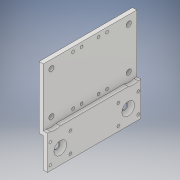
# Autodesk Inventor part: КВ33.044.201
Saved by Autodesk Inventor 2019 (Build 230136000, 136)
## iProperties
Created: 2019-07-15
Part Number: КВ33.044.201
Material: Пластик АБС
Document SubType Name: Modeling
Designer: Петров Иван
Density: 1.06 g/cm^3
Appearance: Гладкий — белый
Description: Щека каретки
Mass: 64.5472 g
Surface Area: 280.738 cm^2
Volume: 60.8936 cm^3
Author: Петров Иван
Autodesk Inventor part; units mm, degrees
(part 1 of 3)
ref_plane "YZ Plane" through (0, 0, 0) normal (1, 0, 0) x (0, 1, 0)
ref_plane "XZ Plane" through (0, 0, 0) normal (0, 1, 0) x (-1, 0, 0)
ref_plane "XY Plane" through (0, 0, 0) normal (0, 0, 1) x (1, 0, 0)
sketch "Эскиз1" plane through (0, 0, 0) normal (1, 0, 0) x (0, 1, 0)
  line L0 (34, 15) -> (34, -15)
  line L1 (-34, -15) -> (-34, 15)
  line L2 (-34, 15) -> (-34, 55)
  line L3 (-34, 55) -> (34, 55)
  line L4 (34, 55) -> (34, 15)
  line L5 (-34, -15) -> (-34, -55)
  line L6 (-34, -55) -> (34, -55)
  line L7 (34, -55) -> (34, -15)
  line L8 (34, 55) -> (24.5, 55)
  line L9 (24.5, 55) -> (24.5, 45.5)
  line L10 (27.5, 45.5) -> (34, 45.5)
  line L11 (34, 45.5) -> (34, 55)
  line L12 (-34, 55) -> (-24.5, 55)
  line L13 (-24.5, 55) -> (-24.5, 45.5)
  line L14 (-27.5, 45.5) -> (-34, 45.5)
  line L15 (-34, 45.5) -> (-34, 55)
  line L16 (-34, -55) -> (-24.5, -55)
  line L17 (-24.5, -55) -> (-24.5, -45.5)
  line L18 (-27.5, -45.5) -> (-34, -45.5)
  line L19 (-34, -45.5) -> (-34, -55)
  line L20 (34, -55) -> (24.5, -55)
  line L21 (24.5, -55) -> (24.5, -45.5)
  line L22 (27.5, -45.5) -> (34, -45.5)
  line L23 (34, -45.5) -> (34, -55)
  circle A0 centre (24.5, 45.5) radius 3
  circle A1 centre (-24.5, 45.5) radius 3
  circle A2 centre (-24.5, -45.5) radius 3
  circle A3 centre (24.5, -45.5) radius 3
  line L24 (34, 55) -> (-34, 55)
  line L25 (-34, 55) -> (-34, -55)
  line L26 (-34, -55) -> (34, -55)
  line L27 (34, -55) -> (34, 55)
  point P0 (0, 0)
  dimension "d12" = 6
  dimension "d13" = 6
  dimension "d14" = 6
  dimension "d15" = 6
  dimension "d4" = 9.5
  dimension "d5" = 9.5
  dimension "d6" = 9.5
  dimension "d7" = 9.5
  dimension "d8" = 9.5
  dimension "d9" = 9.5
  dimension "d10" = 9.5
  dimension "d11" = 9.5
  constraints: 56 end point, 13 parallel, 7 horizontal, 5 perpendicular, 5 vertical, 4 coincident, 4 horizontal alignment, 1 point on line, 8 other
  measures "d4" distance of L10.end L9.end
  measures "d5" distance of L9.end L8.end
  measures "d6" distance of L13.end L14.end
  measures "d7" distance of L12.end L13.end
  measures "d8" distance of L16.end L17.end
  measures "d9" distance of L17.end L18.end
  measures "d10" distance of L20.end L21.end
  measures "d11" distance of L21.end L22.end
extrude "Выдавливание1" add sketch "Эскиз1" along normal blind 5 contours L0 L7 L22 A3 L21 L6 L17 A2 L18 L5 L1 L2 L14 A1 L13 L3 L9 A0 L10 L4 | L10 A0 L9 L3 L4 | L7 L6 L21 A3 L22 | L13 A1 L14 L2 L3 | L6 L5 L18 A2 L17
sketch "Эскиз2" plane through (0, -34, -55) normal (0, -1, 0) x (1, 0, 0)
  line L0 (0, 110) -> (5, 110) projected
  line L1 (0, 110) -> (10, 110)
  line L2 (10, 110) -> (10, 0)
  line L3 (10, 0) -> (0, 0)
  line L4 (0, 0) -> (0, 110)
  point P0 (0, 55)
  dimension "d18" = 10
  dimension "d19" = 110
  constraints: 8 end point, 2 parallel, 1 horizontal, 1 perpendicular
  measures "d18" distance of L2.end L3.end
  measures "d19" distance of L1.end L2.end
extrude "Выдавливание2" add sketch "Эскиз2" along normal blind 5
sketch "Эскиз3" plane through (0, -39, -55) normal (0, -1, 0) x (1, 0, 0)
  line L0 (10, 0) -> (10, 110) projected
  line L1 (5, 0) -> (5, 110) projected
  line L2 (10, 110) -> (5, 110)
  line L3 (5, 110) -> (5, 0)
  line L4 (5, 0) -> (10, 0)
  line L5 (10, 0) -> (10, 110)
  point P0 (0, 55)
  constraints: 8 end point, 2 parallel, 1 horizontal, 1 perpendicular
extrude "Выдавливание3" add sketch "Эскиз3" along normal blind 35
sketch "Эскиз4" plane through (5, -39, -55) normal (-1, 0, 0) x (0, 0, 1)
  arc A0 (18.9646, -11.5001) -> (20.0253, -11.0608) centre (18.9646, -10.0001) ccw
  line L0 (18.9646, -11.5001) -> (15.7747, -11.5001)
  line L1 (15.7747, -11.5001) -> (15.0002, -12.15)
  line L2 (15.0002, -12.15) -> (14.2254, -11.4999)
  line L3 (14.2254, -11.4999) -> (11.0358, -11.4999)
  arc A1 (9.9751, -11.0606) -> (11.0358, -11.4999) centre (11.0358, -9.9999) ccw
  line L4 (9.9751, -11.0606) -> (6.6464, -7.7319)
  arc A2 (6.5, -7.3783) -> (6.6464, -7.7319) centre (7, -7.3783) ccw
  line L5 (6.5, -7.3783) -> (6.5, -4.9)
  arc A3 (6.7, -4.7) -> (6.5, -4.9) centre (6.7, -4.9) ccw
  line L6 (6.7, -4.7) -> (10.7, -4.7)
  arc A4 (10.7, -4.7) -> (10.9, -4.5) centre (10.7, -4.5) ccw
  line L7 (10.9, -4.5) -> (10.9, -3.4)
  arc A5 (10.9, -3.4) -> (10.7, -3.2) centre (10.7, -3.4) ccw
  line L8 (10.7, -3.2) -> (10.3, -3.2)
  line L9 (10.3, -3.2) -> (10.3, -2.6999)
  arc A6 (10.3, -2.6999) -> (10.0999, -2.4999) centre (10.0999, -2.6999) ccw
  line L10 (10.0999, -2.4999) -> (1.5, -2.4999)
  arc A7 (1.5, -2.4999) -> (0, -3.9999) centre (1.5, -3.9999) ccw
  line L11 (0, -3.9999) -> (0, -12.6001)
  arc A8 (0, -12.6001) -> (0.2, -12.8001) centre (0.2, -12.6001) ccw
  line L12 (0.2, -12.8001) -> (0.7, -12.8001)
  line L13 (0.7, -12.8001) -> (0.7, -13.2001)
  arc A9 (0.7, -13.2001) -> (0.9, -13.4001) centre (0.9, -13.2001) ccw
  line L14 (0.9, -13.4001) -> (2, -13.4001)
  arc A10 (2, -13.4001) -> (2.2, -13.2001) centre (2, -13.2001) ccw
  line L15 (2.2, -13.2001) -> (2.2, -9.2)
  arc A11 (2.4, -9) -> (2.2, -9.2) centre (2.4, -9.2) ccw
  line L16 (2.4, -9) -> (4.8789, -9)
  arc A12 (5.2325, -9.1464) -> (4.8789, -9) centre (4.8789, -9.5) ccw
  line L17 (5.2325, -9.1464) -> (8.5608, -12.4747)
  arc A13 (9.0001, -13.5354) -> (8.5608, -12.4747) centre (7.5001, -13.5354) ccw
  line L18 (9.0001, -13.5354) -> (9.0001, -16.7253)
  line L19 (9.0001, -16.7253) -> (9.65, -17.4998)
  line L20 (9.65, -17.4998) -> (8.9999, -18.2746)
  line L21 (8.9999, -18.2746) -> (8.9999, -21.4642)
  arc A14 (8.5606, -22.5249) -> (8.9999, -21.4642) centre (7.4999, -21.4642) ccw
  line L22 (8.5606, -22.5249) -> (5.2319, -25.8536)
  arc A15 (4.8783, -26) -> (5.2319, -25.8536) centre (4.8783, -25.5) ccw
  line L23 (4.8783, -26) -> (2.4, -26)
  arc A16 (2.2, -25.8) -> (2.4, -26) centre (2.4, -25.8) ccw
  line L24 (2.2, -25.8) -> (2.2, -21.8)
  arc A17 (2.2, -21.8) -> (2, -21.6) centre (2, -21.8) ccw
  line L25 (2, -21.6) -> (0.9, -21.6)
  arc A18 (0.9, -21.6) -> (0.7, -21.8) centre (0.9, -21.8) ccw
  line L26 (0.7, -21.8) -> (0.7, -22.2)
  line L27 (0.7, -22.2) -> (0.2, -22.2)
  arc A19 (0.2, -22.2) -> (0, -22.4) centre (0.2, -22.4) ccw
  line L28 (0, -22.4) -> (0, -31)
  arc A20 (0, -31) -> (1.5, -32.5) centre (1.5, -31) ccw
  line L29 (1.5, -32.5) -> (10.1002, -32.5)
  arc A21 (10.1002, -32.5) -> (10.3002, -32.3) centre (10.1002, -32.3) ccw
  line L30 (10.3002, -32.3) -> (10.3002, -31.8)
  line L31 (10.3002, -31.8) -> (10.7002, -31.8)
  arc A22 (10.7002, -31.8) -> (10.9002, -31.6) centre (10.7002, -31.6) ccw
  line L32 (10.9002, -31.6) -> (10.9002, -30.5)
  arc A23 (10.9002, -30.5) -> (10.7002, -30.3) centre (10.7002, -30.5) ccw
  line L33 (10.7002, -30.3) -> (6.7001, -30.3)
  arc A24 (6.5001, -30.1) -> (6.7001, -30.3) centre (6.7001, -30.1) ccw
  line L34 (6.5001, -30.1) -> (6.5001, -27.6211)
  arc A25 (6.6466, -27.2675) -> (6.5001, -27.6211) centre (7.0001, -27.6211) ccw
  line L35 (6.6466, -27.2675) -> (9.9749, -23.9392)
  arc A26 (11.0355, -23.4999) -> (9.9749, -23.9392) centre (11.0355, -24.9999) ccw
  line L36 (11.0355, -23.4999) -> (14.2255, -23.4999)
  line L37 (14.2255, -23.4999) -> (15, -22.85)
  line L38 (15, -22.85) -> (15.7747, -23.5001)
  line L39 (15.7747, -23.5001) -> (18.9644, -23.5001)
  arc A27 (20.025, -23.9394) -> (18.9644, -23.5001) centre (18.9644, -25.0001) ccw
  line L40 (20.025, -23.9394) -> (23.3537, -27.2681)
  arc A28 (23.5001, -27.6217) -> (23.3537, -27.2681) centre (23.0001, -27.6217) ccw
  line L41 (23.5001, -27.6217) -> (23.5001, -30.1)
  arc A29 (23.3001, -30.3) -> (23.5001, -30.1) centre (23.3001, -30.1) ccw
  line L42 (23.3001, -30.3) -> (19.3002, -30.3)
  arc A30 (19.3002, -30.3) -> (19.1002, -30.5) centre (19.3002, -30.5) ccw
  line L43 (19.1002, -30.5) -> (19.1002, -31.6)
  arc A31 (19.1002, -31.6) -> (19.3002, -31.8) centre (19.3002, -31.6) ccw
  line L44 (19.3002, -31.8) -> (19.7002, -31.8)
  line L45 (19.7002, -31.8) -> (19.7002, -32.3)
  arc A32 (19.7002, -32.3) -> (19.9002, -32.5) centre (19.9002, -32.3) ccw
  line L46 (19.9002, -32.5) -> (28.5001, -32.5)
  arc A33 (28.5001, -32.5) -> (30.0001, -31) centre (28.5001, -31) ccw
  line L47 (30.0001, -31) -> (30.0001, -22.3998)
  arc A34 (30.0001, -22.3998) -> (29.8001, -22.1998) centre (29.8001, -22.3998) ccw
  line L48 (29.8001, -22.1998) -> (29.3001, -22.1998)
  line L49 (29.3001, -22.1998) -> (29.3001, -21.7998)
  arc A35 (29.3001, -21.7998) -> (29.1001, -21.5998) centre (29.1001, -21.7998) ccw
  line L50 (29.1001, -21.5998) -> (28.0001, -21.5998)
  arc A36 (28.0001, -21.5998) -> (27.8001, -21.7998) centre (28.0001, -21.7998) ccw
  line L51 (27.8001, -21.7998) -> (27.8001, -25.7999)
  arc A37 (27.6001, -25.9999) -> (27.8001, -25.7999) centre (27.6001, -25.7999) ccw
  line L52 (27.6001, -25.9999) -> (25.1212, -25.9999)
  arc A38 (24.7677, -25.8534) -> (25.1212, -25.9999) centre (25.1212, -25.4999) ccw
  line L53 (24.7677, -25.8534) -> (21.4394, -22.5251)
  arc A39 (21, -21.4645) -> (21.4394, -22.5251) centre (22.5, -21.4645) ccw
  line L54 (21, -21.4645) -> (21, -18.2745)
  line L55 (21, -18.2745) -> (20.3501, -17.5)
  line L56 (20.3501, -17.5) -> (21.0002, -16.7253)
  line L57 (21.0002, -16.7253) -> (21.0002, -13.5356)
  arc A40 (21.4396, -12.475) -> (21.0002, -13.5356) centre (22.5002, -13.5356) ccw
  line L58 (21.4396, -12.475) -> (24.7682, -9.1463)
  arc A41 (25.1218, -8.9999) -> (24.7682, -9.1463) centre (25.1218, -9.4999) ccw
  line L59 (25.1218, -8.9999) -> (27.6001, -8.9999)
  arc A42 (27.8001, -9.1999) -> (27.6001, -8.9999) centre (27.6001, -9.1999) ccw
  line L60 (27.8001, -9.1999) -> (27.8001, -13.1998)
  arc A43 (27.8001, -13.1998) -> (28.0001, -13.3998) centre (28.0001, -13.1998) ccw
  line L61 (28.0001, -13.3998) -> (29.1001, -13.3998)
  arc A44 (29.1001, -13.3998) -> (29.3001, -13.1998) centre (29.1001, -13.1998) ccw
  line L62 (29.3001, -13.1998) -> (29.3001, -12.7999)
  line L63 (29.3001, -12.7999) -> (29.8001, -12.7999)
  arc A45 (29.8001, -12.7999) -> (30.0001, -12.5999) centre (29.8001, -12.5999) ccw
  line L64 (30.0001, -12.5999) -> (30.0001, -3.9998)
  arc A46 (30.0001, -3.9998) -> (28.5001, -2.4998) centre (28.5001, -3.9998) ccw
  line L65 (28.5001, -2.4998) -> (19.8999, -2.4998)
  arc A47 (19.8999, -2.4998) -> (19.6999, -2.6998) centre (19.8999, -2.6998) ccw
  line L66 (19.6999, -2.6998) -> (19.6999, -3.2)
  line L67 (19.6999, -3.2) -> (19.2999, -3.2)
  arc A48 (19.2999, -3.2) -> (19.0999, -3.4) centre (19.2999, -3.4) ccw
  line L68 (19.0999, -3.4) -> (19.0999, -4.5)
  arc A49 (19.0999, -4.5) -> (19.2999, -4.7) centre (19.2999, -4.5) ccw
  line L69 (19.2999, -4.7) -> (23.3, -4.7)
  arc A50 (23.5, -4.9) -> (23.3, -4.7) centre (23.3, -4.9) ccw
  line L70 (23.5, -4.9) -> (23.5, -7.3789)
  arc A51 (23.3536, -7.7325) -> (23.5, -7.3789) centre (23, -7.3789) ccw
  line L71 (23.3536, -7.7325) -> (20.0253, -11.0608)
  arc A52 (2.2887, -27.7413) -> (2.5454, -27.8134) centre (2.4574, -27.6338) ccw
  arc A53 (3.9543, -27.8134) -> (2.5454, -27.8134) centre (3.2499, -29.25) ccw
  arc A54 (3.9543, -27.8134) -> (4.211, -27.7413) centre (4.0423, -27.6338) ccw
  line L72 (4.3695, -27.4925) -> (4.211, -27.7413)
  arc A55 (4.5382, -27.4) -> (4.3695, -27.4925) centre (4.5382, -27.6) ccw
  line L73 (4.6999, -27.4) -> (4.5382, -27.4)
  arc A56 (5.0999, -27.8) -> (4.6999, -27.4) centre (4.6999, -27.8) ccw
  line L74 (5.0999, -27.9617) -> (5.0999, -27.8)
  arc A57 (5.0073, -28.1304) -> (5.0999, -27.9617) centre (4.8999, -27.9617) ccw
  line L75 (4.7586, -28.2888) -> (5.0073, -28.1304)
  arc A58 (4.7586, -28.2888) -> (4.6864, -28.5456) centre (4.866, -28.4575) ccw
  arc A59 (4.6864, -29.9544) -> (4.6864, -28.5456) centre (3.2499, -29.25) ccw
  arc A60 (4.6864, -29.9544) -> (4.7586, -30.2111) centre (4.866, -30.0425) ccw
  line L76 (5.0073, -30.3696) -> (4.7586, -30.2111)
  arc A61 (5.0999, -30.5383) -> (5.0073, -30.3696) centre (4.8999, -30.5383) ccw
  line L77 (5.0999, -30.7) -> (5.0999, -30.5383)
  arc A62 (4.6999, -31.1) -> (5.0999, -30.7) centre (4.6999, -30.7) ccw
  line L78 (4.5382, -31.1) -> (4.6999, -31.1)
  arc A63 (4.3695, -31.0075) -> (4.5382, -31.1) centre (4.5382, -30.9) ccw
  line L79 (4.211, -30.7587) -> (4.3695, -31.0075)
  arc A64 (4.211, -30.7587) -> (3.9543, -30.6866) centre (4.0423, -30.8662) ccw
  arc A65 (2.5454, -30.6866) -> (3.9543, -30.6866) centre (3.2499, -29.25) ccw
  arc A66 (2.5454, -30.6866) -> (2.2887, -30.7587) centre (2.4574, -30.8662) ccw
  line L80 (2.1302, -31.0075) -> (2.2887, -30.7587)
  arc A67 (1.9615, -31.1) -> (2.1302, -31.0075) centre (1.9615, -30.9) ccw
  line L81 (1.7999, -31.1) -> (1.9615, -31.1)
  arc A68 (1.3999, -30.7) -> (1.7999, -31.1) centre (1.7999, -30.7) ccw
  line L82 (1.3999, -30.5383) -> (1.3999, -30.7)
  arc A69 (1.4924, -30.3696) -> (1.3999, -30.5383) centre (1.5999, -30.5383) ccw
  line L83 (1.7411, -30.2111) -> (1.4924, -30.3696)
  arc A70 (1.7411, -30.2111) -> (1.8133, -29.9544) centre (1.6337, -30.0425) ccw
  arc A71 (1.8133, -28.5456) -> (1.8133, -29.9544) centre (3.2499, -29.25) ccw
  arc A72 (1.8133, -28.5456) -> (1.7411, -28.2888) centre (1.6337, -28.4575) ccw
  line L84 (1.4924, -28.1304) -> (1.7411, -28.2888)
  arc A73 (1.3999, -27.9617) -> (1.4924, -28.1304) centre (1.5999, -27.9617) ccw
  line L85 (1.3999, -27.8) -> (1.3999, -27.9617)
  arc A74 (1.7999, -27.4) -> (1.3999, -27.8) centre (1.7999, -27.8) ccw
  line L86 (1.9615, -27.4) -> (1.7999, -27.4)
  arc A75 (2.1302, -27.4925) -> (1.9615, -27.4) centre (1.9615, -27.6) ccw
  line L87 (2.2887, -27.7413) -> (2.1302, -27.4925)
  arc A76 (25.2413, -30.2113) -> (25.3134, -29.9546) centre (25.1338, -30.0426) ccw
  arc A77 (25.3134, -28.5457) -> (25.3134, -29.9546) centre (26.75, -29.2501) ccw
  arc A78 (25.3134, -28.5457) -> (25.2413, -28.289) centre (25.1338, -28.4577) ccw
  line L88 (24.9925, -28.1305) -> (25.2413, -28.289)
  arc A79 (24.9, -27.9618) -> (24.9925, -28.1305) centre (25.1, -27.9618) ccw
  line L89 (24.9, -27.8001) -> (24.9, -27.9618)
  arc A80 (25.3, -27.4001) -> (24.9, -27.8001) centre (25.3, -27.8001) ccw
  line L90 (25.4617, -27.4001) -> (25.3, -27.4001)
  arc A81 (25.6304, -27.4927) -> (25.4617, -27.4001) centre (25.4617, -27.6001) ccw
  line L91 (25.7888, -27.7414) -> (25.6304, -27.4927)
  arc A82 (25.7888, -27.7414) -> (26.0456, -27.8136) centre (25.9575, -27.634) ccw
  arc A83 (27.4544, -27.8136) -> (26.0456, -27.8136) centre (26.75, -29.2501) ccw
  arc A84 (27.4544, -27.8136) -> (27.7111, -27.7414) centre (27.5425, -27.634) ccw
  line L92 (27.8696, -27.4927) -> (27.7111, -27.7414)
  arc A85 (28.0383, -27.4001) -> (27.8696, -27.4927) centre (28.0383, -27.6001) ccw
  line L93 (28.2, -27.4001) -> (28.0383, -27.4001)
  arc A86 (28.6, -27.8001) -> (28.2, -27.4001) centre (28.2, -27.8001) ccw
  line L94 (28.6, -27.9618) -> (28.6, -27.8001)
  arc A87 (28.5075, -28.1305) -> (28.6, -27.9618) centre (28.4, -27.9618) ccw
  line L95 (28.2587, -28.289) -> (28.5075, -28.1305)
  arc A88 (28.2587, -28.289) -> (28.1866, -28.5457) centre (28.3662, -28.4577) ccw
  arc A89 (28.1866, -29.9546) -> (28.1866, -28.5457) centre (26.75, -29.2501) ccw
  arc A90 (28.1866, -29.9546) -> (28.2587, -30.2113) centre (28.3662, -30.0426) ccw
  line L96 (28.5075, -30.3698) -> (28.2587, -30.2113)
  arc A91 (28.6, -30.5385) -> (28.5075, -30.3698) centre (28.4, -30.5385) ccw
  line L97 (28.6, -30.7001) -> (28.6, -30.5385)
  arc A92 (28.2, -31.1001) -> (28.6, -30.7001) centre (28.2, -30.7001) ccw
  line L98 (28.0383, -31.1001) -> (28.2, -31.1001)
  arc A93 (27.8696, -31.0076) -> (28.0383, -31.1001) centre (28.0383, -30.9001) ccw
  line L99 (27.7111, -30.7589) -> (27.8696, -31.0076)
  arc A94 (27.7111, -30.7589) -> (27.4544, -30.6867) centre (27.5425, -30.8663) ccw
  arc A95 (26.0456, -30.6867) -> (27.4544, -30.6867) centre (26.75, -29.2501) ccw
  arc A96 (26.0456, -30.6867) -> (25.7888, -30.7589) centre (25.9575, -30.8663) ccw
  line L100 (25.6304, -31.0076) -> (25.7888, -30.7589)
  arc A97 (25.4617, -31.1001) -> (25.6304, -31.0076) centre (25.4617, -30.9001) ccw
  line L101 (25.3, -31.1001) -> (25.4617, -31.1001)
  arc A98 (24.9, -30.7001) -> (25.3, -31.1001) centre (25.3, -30.7001) ccw
  line L102 (24.9, -30.5385) -> (24.9, -30.7001)
  arc A99 (24.9925, -30.3698) -> (24.9, -30.5385) centre (25.1, -30.5385) ccw
  line L103 (25.2413, -30.2113) -> (24.9925, -30.3698)
  arc A100 (18.1213, -19.0836) -> (18.1996, -19.3473) centre (18.2996, -19.1741) ccw
  line L104 (18.7642, -19.6733) -> (18.1996, -19.3473)
  arc A101 (18.7642, -19.6733) -> (19.0056, -19.6415) centre (18.8642, -19.5001) ccw
  line L105 (19.1586, -19.4885) -> (19.0056, -19.6415)
  arc A102 (19.5, -19.63) -> (19.1586, -19.4885) centre (19.3, -19.63) ccw
  line L106 (19.5, -21) -> (19.5, -19.63)
  arc A103 (18.5, -22) -> (19.5, -21) centre (18.5, -21) ccw
  line L107 (17.13, -22) -> (18.5, -22)
  arc A104 (16.9885, -21.6586) -> (17.13, -22) centre (17.13, -21.8) ccw
  line L108 (17.1415, -21.5056) -> (16.9885, -21.6586)
  arc A105 (17.1415, -21.5056) -> (17.1733, -21.2642) centre (17.0001, -21.3642) ccw
  line L109 (16.8473, -20.6996) -> (17.1733, -21.2642)
  arc A106 (16.8473, -20.6996) -> (16.5836, -20.6213) centre (16.6741, -20.7996) ccw
  arc A107 (13.4164, -20.6213) -> (16.5836, -20.6213) centre (15, -17.5) ccw
  arc A108 (13.4164, -20.6213) -> (13.1527, -20.6996) centre (13.3259, -20.7996) ccw
  line L110 (12.8267, -21.2642) -> (13.1527, -20.6996)
  arc A109 (12.8267, -21.2642) -> (12.8585, -21.5056) centre (12.9999, -21.3642) ccw
  line L111 (13.0115, -21.6586) -> (12.8585, -21.5056)
  arc A110 (12.87, -22) -> (13.0115, -21.6586) centre (12.87, -21.8) ccw
  line L112 (11.5, -22) -> (12.87, -22)
  arc A111 (10.5, -21) -> (11.5, -22) centre (11.5, -21) ccw
  line L113 (10.5, -19.63) -> (10.5, -21)
  arc A112 (10.8414, -19.4885) -> (10.5, -19.63) centre (10.7, -19.63) ccw
  line L114 (10.9944, -19.6415) -> (10.8414, -19.4885)
  arc A113 (10.9944, -19.6415) -> (11.2358, -19.6733) centre (11.1358, -19.5001) ccw
  line L115 (11.8004, -19.3473) -> (11.2358, -19.6733)
  arc A114 (11.8004, -19.3473) -> (11.8787, -19.0836) centre (11.7004, -19.1741) ccw
  arc A115 (11.8787, -15.9164) -> (11.8787, -19.0836) centre (15, -17.5) ccw
  arc A116 (11.8787, -15.9164) -> (11.8004, -15.6527) centre (11.7004, -15.8259) ccw
  line L116 (11.2358, -15.3267) -> (11.8004, -15.6527)
  arc A117 (11.2358, -15.3267) -> (10.9944, -15.3585) centre (11.1358, -15.4999) ccw
  line L117 (10.8414, -15.5115) -> (10.9944, -15.3585)
  arc A118 (10.5, -15.37) -> (10.8414, -15.5115) centre (10.7, -15.37) ccw
  line L118 (10.5, -14) -> (10.5, -15.37)
  arc A119 (11.5, -13) -> (10.5, -14) centre (11.5, -14) ccw
  line L119 (12.87, -13) -> (11.5, -13)
  arc A120 (13.0115, -13.3414) -> (12.87, -13) centre (12.87, -13.2) ccw
  line L120 (12.8585, -13.4944) -> (13.0115, -13.3414)
  arc A121 (12.8585, -13.4944) -> (12.8267, -13.7358) centre (12.9999, -13.6358) ccw
  line L121 (13.1527, -14.3004) -> (12.8267, -13.7358)
  arc A122 (13.1527, -14.3004) -> (13.4164, -14.3787) centre (13.3259, -14.2004) ccw
  arc A123 (16.5836, -14.3787) -> (13.4164, -14.3787) centre (15, -17.5) ccw
  arc A124 (16.5836, -14.3787) -> (16.8473, -14.3004) centre (16.6741, -14.2004) ccw
  line L122 (17.1733, -13.7358) -> (16.8473, -14.3004)
  arc A125 (17.1733, -13.7358) -> (17.1415, -13.4944) centre (17.0001, -13.6358) ccw
  line L123 (16.9885, -13.3414) -> (17.1415, -13.4944)
  arc A126 (17.13, -13) -> (16.9885, -13.3414) centre (17.13, -13.2) ccw
  line L124 (18.5, -13) -> (17.13, -13)
  arc A127 (19.5, -14) -> (18.5, -13) centre (18.5, -14) ccw
  line L125 (19.5, -15.37) -> (19.5, -14)
  arc A128 (19.1586, -15.5115) -> (19.5, -15.37) centre (19.3, -15.37) ccw
  line L126 (19.0056, -15.3585) -> (19.1586, -15.5115)
  arc A129 (19.0056, -15.3585) -> (18.7642, -15.3267) centre (18.8642, -15.4999) ccw
  line L127 (18.1996, -15.6527) -> (18.7642, -15.3267)
  arc A130 (18.1996, -15.6527) -> (18.1213, -15.9164) centre (18.2996, -15.8259) ccw
  arc A131 (18.1213, -19.0836) -> (18.1213, -15.9164) centre (15, -17.5) ccw
  arc A132 (27.7113, -7.2587) -> (27.4546, -7.1866) centre (27.5426, -7.3662) ccw
  arc A133 (26.0457, -7.1866) -> (27.4546, -7.1866) centre (26.7501, -5.75) ccw
  arc A134 (26.0457, -7.1866) -> (25.789, -7.2587) centre (25.9577, -7.3662) ccw
  line L128 (25.6305, -7.5075) -> (25.789, -7.2587)
  arc A135 (25.4618, -7.6) -> (25.6305, -7.5075) centre (25.4618, -7.4) ccw
  line L129 (25.3001, -7.6) -> (25.4618, -7.6)
  arc A136 (24.9001, -7.2) -> (25.3001, -7.6) centre (25.3001, -7.2) ccw
  line L130 (24.9001, -7.0383) -> (24.9001, -7.2)
  arc A137 (24.9927, -6.8696) -> (24.9001, -7.0383) centre (25.1001, -7.0383) ccw
  line L131 (25.2414, -6.7112) -> (24.9927, -6.8696)
  arc A138 (25.2414, -6.7112) -> (25.3136, -6.4544) centre (25.134, -6.5425) ccw
  arc A139 (25.3136, -5.0456) -> (25.3136, -6.4544) centre (26.7501, -5.75) ccw
  arc A140 (25.3136, -5.0456) -> (25.2414, -4.7889) centre (25.134, -4.9575) ccw
  line L132 (24.9927, -4.6304) -> (25.2414, -4.7889)
  arc A141 (24.9001, -4.4617) -> (24.9927, -4.6304) centre (25.1001, -4.4617) ccw
  line L133 (24.9001, -4.3) -> (24.9001, -4.4617)
  arc A142 (25.3001, -3.9) -> (24.9001, -4.3) centre (25.3001, -4.3) ccw
  line L134 (25.4618, -3.9) -> (25.3001, -3.9)
  arc A143 (25.6305, -3.9925) -> (25.4618, -3.9) centre (25.4618, -4.1) ccw
  line L135 (25.789, -4.2413) -> (25.6305, -3.9925)
  arc A144 (25.789, -4.2413) -> (26.0457, -4.3134) centre (25.9577, -4.1338) ccw
  arc A145 (27.4546, -4.3134) -> (26.0457, -4.3134) centre (26.7501, -5.75) ccw
  arc A146 (27.4546, -4.3134) -> (27.7113, -4.2413) centre (27.5426, -4.1338) ccw
  line L136 (27.8698, -3.9925) -> (27.7113, -4.2413)
  arc A147 (28.0385, -3.9) -> (27.8698, -3.9925) centre (28.0385, -4.1) ccw
  line L137 (28.2001, -3.9) -> (28.0385, -3.9)
  arc A148 (28.6001, -4.3) -> (28.2001, -3.9) centre (28.2001, -4.3) ccw
  line L138 (28.6001, -4.4617) -> (28.6001, -4.3)
  arc A149 (28.5076, -4.6304) -> (28.6001, -4.4617) centre (28.4001, -4.4617) ccw
  line L139 (28.2589, -4.7889) -> (28.5076, -4.6304)
  arc A150 (28.2589, -4.7889) -> (28.1867, -5.0456) centre (28.3663, -4.9575) ccw
  arc A151 (28.1867, -6.4544) -> (28.1867, -5.0456) centre (26.7501, -5.75) ccw
  arc A152 (28.1867, -6.4544) -> (28.2589, -6.7112) centre (28.3663, -6.5425) ccw
  line L140 (28.5076, -6.8696) -> (28.2589, -6.7112)
  arc A153 (28.6001, -7.0383) -> (28.5076, -6.8696) centre (28.4001, -7.0383) ccw
  line L141 (28.6001, -7.2) -> (28.6001, -7.0383)
  arc A154 (28.2001, -7.6) -> (28.6001, -7.2) centre (28.2001, -7.2) ccw
  line L142 (28.0385, -7.6) -> (28.2001, -7.6)
  arc A155 (27.8698, -7.5075) -> (28.0385, -7.6) centre (28.0385, -7.4) ccw
  line L143 (27.7113, -7.2587) -> (27.8698, -7.5075)
  arc A156 (4.7587, -4.7887) -> (4.6866, -5.0454) centre (4.8662, -4.9574) ccw
  arc A157 (4.6866, -6.4543) -> (4.6866, -5.0454) centre (3.25, -5.7499) ccw
  arc A158 (4.6866, -6.4543) -> (4.7587, -6.711) centre (4.8662, -6.5423) ccw
  line L144 (5.0075, -6.8695) -> (4.7587, -6.711)
  arc A159 (5.1, -7.0382) -> (5.0075, -6.8695) centre (4.9, -7.0382) ccw
  line L145 (5.1, -7.1999) -> (5.1, -7.0382)
  arc A160 (4.7, -7.5999) -> (5.1, -7.1999) centre (4.7, -7.1999) ccw
  line L146 (4.5383, -7.5999) -> (4.7, -7.5999)
  arc A161 (4.3696, -7.5073) -> (4.5383, -7.5999) centre (4.5383, -7.3999) ccw
  line L147 (4.2112, -7.2586) -> (4.3696, -7.5073)
  arc A162 (4.2112, -7.2586) -> (3.9544, -7.1864) centre (4.0425, -7.366) ccw
  arc A163 (2.5456, -7.1864) -> (3.9544, -7.1864) centre (3.25, -5.7499) ccw
  arc A164 (2.5456, -7.1864) -> (2.2889, -7.2586) centre (2.4575, -7.366) ccw
  line L148 (2.1304, -7.5073) -> (2.2889, -7.2586)
  arc A165 (1.9617, -7.5999) -> (2.1304, -7.5073) centre (1.9617, -7.3999) ccw
  line L149 (1.8, -7.5999) -> (1.9617, -7.5999)
  arc A166 (1.4, -7.1999) -> (1.8, -7.5999) centre (1.8, -7.1999) ccw
  line L150 (1.4, -7.0382) -> (1.4, -7.1999)
  arc A167 (1.4925, -6.8695) -> (1.4, -7.0382) centre (1.6, -7.0382) ccw
  line L151 (1.7413, -6.711) -> (1.4925, -6.8695)
  arc A168 (1.7413, -6.711) -> (1.8134, -6.4543) centre (1.6338, -6.5423) ccw
  arc A169 (1.8134, -5.0454) -> (1.8134, -6.4543) centre (3.25, -5.7499) ccw
  arc A170 (1.8134, -5.0454) -> (1.7413, -4.7887) centre (1.6338, -4.9574) ccw
  line L152 (1.4925, -4.6302) -> (1.7413, -4.7887)
  arc A171 (1.4, -4.4615) -> (1.4925, -4.6302) centre (1.6, -4.4615) ccw
  line L153 (1.4, -4.2999) -> (1.4, -4.4615)
  arc A172 (1.8, -3.8999) -> (1.4, -4.2999) centre (1.8, -4.2999) ccw
  line L154 (1.9617, -3.8999) -> (1.8, -3.8999)
  arc A173 (2.1304, -3.9924) -> (1.9617, -3.8999) centre (1.9617, -4.0999) ccw
  line L155 (2.2889, -4.2411) -> (2.1304, -3.9924)
  arc A174 (2.2889, -4.2411) -> (2.5456, -4.3133) centre (2.4575, -4.1337) ccw
  arc A175 (3.9544, -4.3133) -> (2.5456, -4.3133) centre (3.25, -5.7499) ccw
  arc A176 (3.9544, -4.3133) -> (4.2112, -4.2411) centre (4.0425, -4.1337) ccw
  line L156 (4.3696, -3.9924) -> (4.2112, -4.2411)
  arc A177 (4.5383, -3.8999) -> (4.3696, -3.9924) centre (4.5383, -4.0999) ccw
  line L157 (4.7, -3.8999) -> (4.5383, -3.8999)
  arc A178 (5.1, -4.2999) -> (4.7, -3.8999) centre (4.7, -4.2999) ccw
  line L158 (5.1, -4.4615) -> (5.1, -4.2999)
  arc A179 (5.0075, -4.6302) -> (5.1, -4.4615) centre (4.9, -4.4615) ccw
  line L159 (4.7587, -4.7887) -> (5.0075, -4.6302)
  line L160 (0, 0) -> (110, 0) projected
  line L161 (55, 0) -> (55, -35)
  line L162 (55, 0) -> (90, 0) construction
  line L163 (55, -17.5) -> (0, -17.5)
  line L164 (0, 5) -> (0, -35) projected
  line L165 (0, -17.5) -> (15, -17.5)
  circle A180 centre (26.7501, -5.75) radius 1.6
  circle A181 centre (26.75, -29.2501) radius 1.6
  circle A182 centre (3.2499, -29.25) radius 1.6
  circle A183 centre (3.25, -5.7499) radius 1.6
  circle A184 centre (15, -17.5) radius 3.5
  arc A185 (89.9747, -11.0608) -> (91.0354, -11.5001) centre (91.0354, -10.0001) ccw
  line L166 (91.0354, -11.5001) -> (94.2253, -11.5001)
  line L167 (94.2253, -11.5001) -> (94.9998, -12.15)
  line L168 (94.9998, -12.15) -> (95.7746, -11.4999)
  line L169 (95.7746, -11.4999) -> (98.9642, -11.4999)
  arc A186 (98.9642, -11.4999) -> (100.0249, -11.0606) centre (98.9642, -9.9999) ccw
  line L170 (100.0249, -11.0606) -> (103.3536, -7.7319)
  arc A187 (103.3536, -7.7319) -> (103.5, -7.3783) centre (103, -7.3783) ccw
  line L171 (103.5, -7.3783) -> (103.5, -4.9)
  arc A188 (103.5, -4.9) -> (103.3, -4.7) centre (103.3, -4.9) ccw
  line L172 (103.3, -4.7) -> (99.3, -4.7)
  arc A189 (99.1, -4.5) -> (99.3, -4.7) centre (99.3, -4.5) ccw
  line L173 (99.1, -4.5) -> (99.1, -3.4)
  arc A190 (99.3, -3.2) -> (99.1, -3.4) centre (99.3, -3.4) ccw
  line L174 (99.3, -3.2) -> (99.7, -3.2)
  line L175 (99.7, -3.2) -> (99.7, -2.6999)
  arc A191 (99.9001, -2.4999) -> (99.7, -2.6999) centre (99.9001, -2.6999) ccw
  line L176 (99.9001, -2.4999) -> (108.5, -2.4999)
  arc A192 (110, -3.9999) -> (108.5, -2.4999) centre (108.5, -3.9999) ccw
  line L177 (110, -3.9999) -> (110, -12.6001)
  arc A193 (109.8, -12.8001) -> (110, -12.6001) centre (109.8, -12.6001) ccw
  line L178 (109.8, -12.8001) -> (109.3, -12.8001)
  line L179 (109.3, -12.8001) -> (109.3, -13.2001)
  arc A194 (109.1, -13.4001) -> (109.3, -13.2001) centre (109.1, -13.2001) ccw
  line L180 (109.1, -13.4001) -> (108, -13.4001)
  arc A195 (107.8, -13.2001) -> (108, -13.4001) centre (108, -13.2001) ccw
  line L181 (107.8, -13.2001) -> (107.8, -9.2)
  arc A196 (107.8, -9.2) -> (107.6, -9) centre (107.6, -9.2) ccw
  line L182 (107.6, -9) -> (105.1211, -9)
  arc A197 (105.1211, -9) -> (104.7675, -9.1464) centre (105.1211, -9.5) ccw
  line L183 (104.7675, -9.1464) -> (101.4392, -12.4747)
  arc A198 (101.4392, -12.4747) -> (100.9999, -13.5354) centre (102.4999, -13.5354) ccw
  line L184 (100.9999, -13.5354) -> (100.9999, -16.7253)
  line L185 (100.9999, -16.7253) -> (100.35, -17.4998)
  line L186 (100.35, -17.4998) -> (101.0001, -18.2746)
  line L187 (101.0001, -18.2746) -> (101.0001, -21.4642)
  arc A199 (101.0001, -21.4642) -> (101.4394, -22.5249) centre (102.5001, -21.4642) ccw
  line L188 (101.4394, -22.5249) -> (104.7681, -25.8536)
  arc A200 (104.7681, -25.8536) -> (105.1217, -26) centre (105.1217, -25.5) ccw
  line L189 (105.1217, -26) -> (107.6, -26)
  arc A201 (107.6, -26) -> (107.8, -25.8) centre (107.6, -25.8) ccw
  line L190 (107.8, -25.8) -> (107.8, -21.8)
  arc A202 (108, -21.6) -> (107.8, -21.8) centre (108, -21.8) ccw
  line L191 (108, -21.6) -> (109.1, -21.6)
  arc A203 (109.3, -21.8) -> (109.1, -21.6) centre (109.1, -21.8) ccw
  line L192 (109.3, -21.8) -> (109.3, -22.2)
  line L193 (109.3, -22.2) -> (109.8, -22.2)
  arc A204 (110, -22.4) -> (109.8, -22.2) centre (109.8, -22.4) ccw
  line L194 (110, -22.4) -> (110, -31)
  arc A205 (108.5, -32.5) -> (110, -31) centre (108.5, -31) ccw
  line L195 (108.5, -32.5) -> (99.8998, -32.5)
  arc A206 (99.6998, -32.3) -> (99.8998, -32.5) centre (99.8998, -32.3) ccw
  line L196 (99.6998, -32.3) -> (99.6998, -31.8)
  line L197 (99.6998, -31.8) -> (99.2998, -31.8)
  arc A207 (99.0998, -31.6) -> (99.2998, -31.8) centre (99.2998, -31.6) ccw
  line L198 (99.0998, -31.6) -> (99.0998, -30.5)
  arc A208 (99.2998, -30.3) -> (99.0998, -30.5) centre (99.2998, -30.5) ccw
  line L199 (99.2998, -30.3) -> (103.2999, -30.3)
  arc A209 (103.2999, -30.3) -> (103.4999, -30.1) centre (103.2999, -30.1) ccw
  line L200 (103.4999, -30.1) -> (103.4999, -27.6211)
  arc A210 (103.4999, -27.6211) -> (103.3534, -27.2675) centre (102.9999, -27.6211) ccw
  line L201 (103.3534, -27.2675) -> (100.0251, -23.9392)
  arc A211 (100.0251, -23.9392) -> (98.9645, -23.4999) centre (98.9645, -24.9999) ccw
  line L202 (98.9645, -23.4999) -> (95.7745, -23.4999)
  line L203 (95.7745, -23.4999) -> (95, -22.85)
  line L204 (95, -22.85) -> (94.2253, -23.5001)
  line L205 (94.2253, -23.5001) -> (91.0356, -23.5001)
  arc A212 (91.0356, -23.5001) -> (89.975, -23.9394) centre (91.0356, -25.0001) ccw
  line L206 (89.975, -23.9394) -> (86.6463, -27.2681)
  arc A213 (86.6463, -27.2681) -> (86.4999, -27.6217) centre (86.9999, -27.6217) ccw
  line L207 (86.4999, -27.6217) -> (86.4999, -30.1)
  arc A214 (86.4999, -30.1) -> (86.6999, -30.3) centre (86.6999, -30.1) ccw
  line L208 (86.6999, -30.3) -> (90.6998, -30.3)
  arc A215 (90.8998, -30.5) -> (90.6998, -30.3) centre (90.6998, -30.5) ccw
  line L209 (90.8998, -30.5) -> (90.8998, -31.6)
  arc A216 (90.6998, -31.8) -> (90.8998, -31.6) centre (90.6998, -31.6) ccw
  line L210 (90.6998, -31.8) -> (90.2998, -31.8)
  line L211 (90.2998, -31.8) -> (90.2998, -32.3)
  arc A217 (90.0998, -32.5) -> (90.2998, -32.3) centre (90.0998, -32.3) ccw
  line L212 (90.0998, -32.5) -> (81.4999, -32.5)
  arc A218 (79.9999, -31) -> (81.4999, -32.5) centre (81.4999, -31) ccw
  line L213 (79.9999, -31) -> (79.9999, -22.3998)
  arc A219 (80.1999, -22.1998) -> (79.9999, -22.3998) centre (80.1999, -22.3998) ccw
  line L214 (80.1999, -22.1998) -> (80.6999, -22.1998)
  line L215 (80.6999, -22.1998) -> (80.6999, -21.7998)
  arc A220 (80.8999, -21.5998) -> (80.6999, -21.7998) centre (80.8999, -21.7998) ccw
  line L216 (80.8999, -21.5998) -> (81.9999, -21.5998)
  arc A221 (82.1999, -21.7998) -> (81.9999, -21.5998) centre (81.9999, -21.7998) ccw
  line L217 (82.1999, -21.7998) -> (82.1999, -25.7999)
  arc A222 (82.1999, -25.7999) -> (82.3999, -25.9999) centre (82.3999, -25.7999) ccw
  line L218 (82.3999, -25.9999) -> (84.8788, -25.9999)
  arc A223 (84.8788, -25.9999) -> (85.2323, -25.8534) centre (84.8788, -25.4999) ccw
  line L219 (85.2323, -25.8534) -> (88.5606, -22.5251)
  arc A224 (88.5606, -22.5251) -> (89, -21.4645) centre (87.5, -21.4645) ccw
  line L220 (89, -21.4645) -> (89, -18.2745)
  line L221 (89, -18.2745) -> (89.6499, -17.5)
  line L222 (89.6499, -17.5) -> (88.9998, -16.7253)
  line L223 (88.9998, -16.7253) -> (88.9998, -13.5356)
  arc A225 (88.9998, -13.5356) -> (88.5604, -12.475) centre (87.4998, -13.5356) ccw
  line L224 (88.5604, -12.475) -> (85.2318, -9.1463)
  arc A226 (85.2318, -9.1463) -> (84.8782, -8.9999) centre (84.8782, -9.4999) ccw
  line L225 (84.8782, -8.9999) -> (82.3999, -8.9999)
  arc A227 (82.3999, -8.9999) -> (82.1999, -9.1999) centre (82.3999, -9.1999) ccw
  line L226 (82.1999, -9.1999) -> (82.1999, -13.1998)
  arc A228 (81.9999, -13.3998) -> (82.1999, -13.1998) centre (81.9999, -13.1998) ccw
  line L227 (81.9999, -13.3998) -> (80.8999, -13.3998)
  arc A229 (80.6999, -13.1998) -> (80.8999, -13.3998) centre (80.8999, -13.1998) ccw
  line L228 (80.6999, -13.1998) -> (80.6999, -12.7999)
  line L229 (80.6999, -12.7999) -> (80.1999, -12.7999)
  arc A230 (79.9999, -12.5999) -> (80.1999, -12.7999) centre (80.1999, -12.5999) ccw
  line L230 (79.9999, -12.5999) -> (79.9999, -3.9998)
  arc A231 (81.4999, -2.4998) -> (79.9999, -3.9998) centre (81.4999, -3.9998) ccw
  line L231 (81.4999, -2.4998) -> (90.1001, -2.4998)
  arc A232 (90.3001, -2.6998) -> (90.1001, -2.4998) centre (90.1001, -2.6998) ccw
  line L232 (90.3001, -2.6998) -> (90.3001, -3.2)
  line L233 (90.3001, -3.2) -> (90.7001, -3.2)
  arc A233 (90.9001, -3.4) -> (90.7001, -3.2) centre (90.7001, -3.4) ccw
  line L234 (90.9001, -3.4) -> (90.9001, -4.5)
  arc A234 (90.7001, -4.7) -> (90.9001, -4.5) centre (90.7001, -4.5) ccw
  line L235 (90.7001, -4.7) -> (86.7, -4.7)
  arc A235 (86.7, -4.7) -> (86.5, -4.9) centre (86.7, -4.9) ccw
  line L236 (86.5, -4.9) -> (86.5, -7.3789)
  arc A236 (86.5, -7.3789) -> (86.6464, -7.7325) centre (87, -7.3789) ccw
  line L237 (86.6464, -7.7325) -> (89.9747, -11.0608)
  arc A237 (107.4546, -27.8134) -> (107.7113, -27.7413) centre (107.5426, -27.6338) ccw
  arc A238 (107.4546, -27.8134) -> (106.0457, -27.8134) centre (106.7501, -29.25) ccw
  arc A239 (105.789, -27.7413) -> (106.0457, -27.8134) centre (105.9577, -27.6338) ccw
  line L238 (105.6305, -27.4925) -> (105.789, -27.7413)
  arc A240 (105.6305, -27.4925) -> (105.4618, -27.4) centre (105.4618, -27.6) ccw
  line L239 (105.3001, -27.4) -> (105.4618, -27.4)
  arc A241 (105.3001, -27.4) -> (104.9001, -27.8) centre (105.3001, -27.8) ccw
  line L240 (104.9001, -27.9617) -> (104.9001, -27.8)
  arc A242 (104.9001, -27.9617) -> (104.9927, -28.1304) centre (105.1001, -27.9617) ccw
  line L241 (105.2414, -28.2888) -> (104.9927, -28.1304)
  arc A243 (105.3136, -28.5456) -> (105.2414, -28.2888) centre (105.134, -28.4575) ccw
  arc A244 (105.3136, -28.5456) -> (105.3136, -29.9544) centre (106.7501, -29.25) ccw
  arc A245 (105.2414, -30.2111) -> (105.3136, -29.9544) centre (105.134, -30.0425) ccw
  line L242 (104.9927, -30.3696) -> (105.2414, -30.2111)
  arc A246 (104.9927, -30.3696) -> (104.9001, -30.5383) centre (105.1001, -30.5383) ccw
  line L243 (104.9001, -30.7) -> (104.9001, -30.5383)
  arc A247 (104.9001, -30.7) -> (105.3001, -31.1) centre (105.3001, -30.7) ccw
  line L244 (105.4618, -31.1) -> (105.3001, -31.1)
  arc A248 (105.4618, -31.1) -> (105.6305, -31.0075) centre (105.4618, -30.9) ccw
  line L245 (105.789, -30.7587) -> (105.6305, -31.0075)
  arc A249 (106.0457, -30.6866) -> (105.789, -30.7587) centre (105.9577, -30.8662) ccw
  arc A250 (106.0457, -30.6866) -> (107.4546, -30.6866) centre (106.7501, -29.25) ccw
  arc A251 (107.7113, -30.7587) -> (107.4546, -30.6866) centre (107.5426, -30.8662) ccw
  line L246 (107.8698, -31.0075) -> (107.7113, -30.7587)
  arc A252 (107.8698, -31.0075) -> (108.0385, -31.1) centre (108.0385, -30.9) ccw
  line L247 (108.2001, -31.1) -> (108.0385, -31.1)
  arc A253 (108.2001, -31.1) -> (108.6001, -30.7) centre (108.2001, -30.7) ccw
  line L248 (108.6001, -30.5383) -> (108.6001, -30.7)
  arc A254 (108.6001, -30.5383) -> (108.5076, -30.3696) centre (108.4001, -30.5383) ccw
  line L249 (108.2589, -30.2111) -> (108.5076, -30.3696)
  arc A255 (108.1867, -29.9544) -> (108.2589, -30.2111) centre (108.3663, -30.0425) ccw
  arc A256 (108.1867, -29.9544) -> (108.1867, -28.5456) centre (106.7501, -29.25) ccw
  arc A257 (108.2589, -28.2888) -> (108.1867, -28.5456) centre (108.3663, -28.4575) ccw
  line L250 (108.5076, -28.1304) -> (108.2589, -28.2888)
  arc A258 (108.5076, -28.1304) -> (108.6001, -27.9617) centre (108.4001, -27.9617) ccw
  line L251 (108.6001, -27.8) -> (108.6001, -27.9617)
  arc A259 (108.6001, -27.8) -> (108.2001, -27.4) centre (108.2001, -27.8) ccw
  line L252 (108.0385, -27.4) -> (108.2001, -27.4)
  arc A260 (108.0385, -27.4) -> (107.8698, -27.4925) centre (108.0385, -27.6) ccw
  line L253 (107.7113, -27.7413) -> (107.8698, -27.4925)
  arc A261 (84.6866, -29.9546) -> (84.7587, -30.2113) centre (84.8662, -30.0426) ccw
  arc A262 (84.6866, -29.9546) -> (84.6866, -28.5457) centre (83.25, -29.2501) ccw
  arc A263 (84.7587, -28.289) -> (84.6866, -28.5457) centre (84.8662, -28.4577) ccw
  line L254 (85.0075, -28.1305) -> (84.7587, -28.289)
  arc A264 (85.0075, -28.1305) -> (85.1, -27.9618) centre (84.9, -27.9618) ccw
  line L255 (85.1, -27.8001) -> (85.1, -27.9618)
  arc A265 (85.1, -27.8001) -> (84.7, -27.4001) centre (84.7, -27.8001) ccw
  line L256 (84.5383, -27.4001) -> (84.7, -27.4001)
  arc A266 (84.5383, -27.4001) -> (84.3696, -27.4927) centre (84.5383, -27.6001) ccw
  line L257 (84.2112, -27.7414) -> (84.3696, -27.4927)
  arc A267 (83.9544, -27.8136) -> (84.2112, -27.7414) centre (84.0425, -27.634) ccw
  arc A268 (83.9544, -27.8136) -> (82.5456, -27.8136) centre (83.25, -29.2501) ccw
  arc A269 (82.2889, -27.7414) -> (82.5456, -27.8136) centre (82.4575, -27.634) ccw
  line L258 (82.1304, -27.4927) -> (82.2889, -27.7414)
  arc A270 (82.1304, -27.4927) -> (81.9617, -27.4001) centre (81.9617, -27.6001) ccw
  line L259 (81.8, -27.4001) -> (81.9617, -27.4001)
  arc A271 (81.8, -27.4001) -> (81.4, -27.8001) centre (81.8, -27.8001) ccw
  line L260 (81.4, -27.9618) -> (81.4, -27.8001)
  arc A272 (81.4, -27.9618) -> (81.4925, -28.1305) centre (81.6, -27.9618) ccw
  line L261 (81.7413, -28.289) -> (81.4925, -28.1305)
  arc A273 (81.8134, -28.5457) -> (81.7413, -28.289) centre (81.6338, -28.4577) ccw
  arc A274 (81.8134, -28.5457) -> (81.8134, -29.9546) centre (83.25, -29.2501) ccw
  arc A275 (81.7413, -30.2113) -> (81.8134, -29.9546) centre (81.6338, -30.0426) ccw
  line L262 (81.4925, -30.3698) -> (81.7413, -30.2113)
  arc A276 (81.4925, -30.3698) -> (81.4, -30.5385) centre (81.6, -30.5385) ccw
  line L263 (81.4, -30.7001) -> (81.4, -30.5385)
  arc A277 (81.4, -30.7001) -> (81.8, -31.1001) centre (81.8, -30.7001) ccw
  line L264 (81.9617, -31.1001) -> (81.8, -31.1001)
  arc A278 (81.9617, -31.1001) -> (82.1304, -31.0076) centre (81.9617, -30.9001) ccw
  line L265 (82.2889, -30.7589) -> (82.1304, -31.0076)
  arc A279 (82.5456, -30.6867) -> (82.2889, -30.7589) centre (82.4575, -30.8663) ccw
  arc A280 (82.5456, -30.6867) -> (83.9544, -30.6867) centre (83.25, -29.2501) ccw
  arc A281 (84.2112, -30.7589) -> (83.9544, -30.6867) centre (84.0425, -30.8663) ccw
  line L266 (84.3696, -31.0076) -> (84.2112, -30.7589)
  arc A282 (84.3696, -31.0076) -> (84.5383, -31.1001) centre (84.5383, -30.9001) ccw
  line L267 (84.7, -31.1001) -> (84.5383, -31.1001)
  arc A283 (84.7, -31.1001) -> (85.1, -30.7001) centre (84.7, -30.7001) ccw
  line L268 (85.1, -30.5385) -> (85.1, -30.7001)
  arc A284 (85.1, -30.5385) -> (85.0075, -30.3698) centre (84.9, -30.5385) ccw
  line L269 (84.7587, -30.2113) -> (85.0075, -30.3698)
  arc A285 (91.8004, -19.3473) -> (91.8787, -19.0836) centre (91.7004, -19.1741) ccw
  line L270 (91.2358, -19.6733) -> (91.8004, -19.3473)
  arc A286 (90.9944, -19.6415) -> (91.2358, -19.6733) centre (91.1358, -19.5001) ccw
  line L271 (90.8414, -19.4885) -> (90.9944, -19.6415)
  arc A287 (90.8414, -19.4885) -> (90.5, -19.63) centre (90.7, -19.63) ccw
  line L272 (90.5, -21) -> (90.5, -19.63)
  arc A288 (90.5, -21) -> (91.5, -22) centre (91.5, -21) ccw
  line L273 (92.87, -22) -> (91.5, -22)
  arc A289 (92.87, -22) -> (93.0115, -21.6586) centre (92.87, -21.8) ccw
  line L274 (92.8585, -21.5056) -> (93.0115, -21.6586)
  arc A290 (92.8267, -21.2642) -> (92.8585, -21.5056) centre (92.9999, -21.3642) ccw
  line L275 (93.1527, -20.6996) -> (92.8267, -21.2642)
  arc A291 (93.4164, -20.6213) -> (93.1527, -20.6996) centre (93.3259, -20.7996) ccw
  arc A292 (93.4164, -20.6213) -> (96.5836, -20.6213) centre (95, -17.5) ccw
  arc A293 (96.8473, -20.6996) -> (96.5836, -20.6213) centre (96.6741, -20.7996) ccw
  line L276 (97.1733, -21.2642) -> (96.8473, -20.6996)
  arc A294 (97.1415, -21.5056) -> (97.1733, -21.2642) centre (97.0001, -21.3642) ccw
  line L277 (96.9885, -21.6586) -> (97.1415, -21.5056)
  arc A295 (96.9885, -21.6586) -> (97.13, -22) centre (97.13, -21.8) ccw
  line L278 (98.5, -22) -> (97.13, -22)
  arc A296 (98.5, -22) -> (99.5, -21) centre (98.5, -21) ccw
  line L279 (99.5, -19.63) -> (99.5, -21)
  arc A297 (99.5, -19.63) -> (99.1586, -19.4885) centre (99.3, -19.63) ccw
  line L280 (99.0056, -19.6415) -> (99.1586, -19.4885)
  arc A298 (98.7642, -19.6733) -> (99.0056, -19.6415) centre (98.8642, -19.5001) ccw
  line L281 (98.1996, -19.3473) -> (98.7642, -19.6733)
  arc A299 (98.1213, -19.0836) -> (98.1996, -19.3473) centre (98.2996, -19.1741) ccw
  arc A300 (98.1213, -19.0836) -> (98.1213, -15.9164) centre (95, -17.5) ccw
  arc A301 (98.1996, -15.6527) -> (98.1213, -15.9164) centre (98.2996, -15.8259) ccw
  line L282 (98.7642, -15.3267) -> (98.1996, -15.6527)
  arc A302 (99.0056, -15.3585) -> (98.7642, -15.3267) centre (98.8642, -15.4999) ccw
  line L283 (99.1586, -15.5115) -> (99.0056, -15.3585)
  arc A303 (99.1586, -15.5115) -> (99.5, -15.37) centre (99.3, -15.37) ccw
  line L284 (99.5, -14) -> (99.5, -15.37)
  arc A304 (99.5, -14) -> (98.5, -13) centre (98.5, -14) ccw
  line L285 (97.13, -13) -> (98.5, -13)
  arc A305 (97.13, -13) -> (96.9885, -13.3414) centre (97.13, -13.2) ccw
  line L286 (97.1415, -13.4944) -> (96.9885, -13.3414)
  arc A306 (97.1733, -13.7358) -> (97.1415, -13.4944) centre (97.0001, -13.6358) ccw
  line L287 (96.8473, -14.3004) -> (97.1733, -13.7358)
  arc A307 (96.5836, -14.3787) -> (96.8473, -14.3004) centre (96.6741, -14.2004) ccw
  arc A308 (96.5836, -14.3787) -> (93.4164, -14.3787) centre (95, -17.5) ccw
  arc A309 (93.1527, -14.3004) -> (93.4164, -14.3787) centre (93.3259, -14.2004) ccw
  line L288 (92.8267, -13.7358) -> (93.1527, -14.3004)
  arc A310 (92.8585, -13.4944) -> (92.8267, -13.7358) centre (92.9999, -13.6358) ccw
  line L289 (93.0115, -13.3414) -> (92.8585, -13.4944)
  arc A311 (93.0115, -13.3414) -> (92.87, -13) centre (92.87, -13.2) ccw
  line L290 (91.5, -13) -> (92.87, -13)
  arc A312 (91.5, -13) -> (90.5, -14) centre (91.5, -14) ccw
  line L291 (90.5, -15.37) -> (90.5, -14)
  arc A313 (90.5, -15.37) -> (90.8414, -15.5115) centre (90.7, -15.37) ccw
  line L292 (90.9944, -15.3585) -> (90.8414, -15.5115)
  arc A314 (91.2358, -15.3267) -> (90.9944, -15.3585) centre (91.1358, -15.4999) ccw
  line L293 (91.8004, -15.6527) -> (91.2358, -15.3267)
  arc A315 (91.8787, -15.9164) -> (91.8004, -15.6527) centre (91.7004, -15.8259) ccw
  arc A316 (91.8787, -15.9164) -> (91.8787, -19.0836) centre (95, -17.5) ccw
  arc A317 (82.5454, -7.1866) -> (82.2887, -7.2587) centre (82.4574, -7.3662) ccw
  arc A318 (82.5454, -7.1866) -> (83.9543, -7.1866) centre (83.2499, -5.75) ccw
  arc A319 (84.211, -7.2587) -> (83.9543, -7.1866) centre (84.0423, -7.3662) ccw
  line L294 (84.3695, -7.5075) -> (84.211, -7.2587)
  arc A320 (84.3695, -7.5075) -> (84.5382, -7.6) centre (84.5382, -7.4) ccw
  line L295 (84.6999, -7.6) -> (84.5382, -7.6)
  arc A321 (84.6999, -7.6) -> (85.0999, -7.2) centre (84.6999, -7.2) ccw
  line L296 (85.0999, -7.0383) -> (85.0999, -7.2)
  arc A322 (85.0999, -7.0383) -> (85.0073, -6.8696) centre (84.8999, -7.0383) ccw
  line L297 (84.7586, -6.7112) -> (85.0073, -6.8696)
  arc A323 (84.6864, -6.4544) -> (84.7586, -6.7112) centre (84.866, -6.5425) ccw
  arc A324 (84.6864, -6.4544) -> (84.6864, -5.0456) centre (83.2499, -5.75) ccw
  arc A325 (84.7586, -4.7889) -> (84.6864, -5.0456) centre (84.866, -4.9575) ccw
  line L298 (85.0073, -4.6304) -> (84.7586, -4.7889)
  arc A326 (85.0073, -4.6304) -> (85.0999, -4.4617) centre (84.8999, -4.4617) ccw
  line L299 (85.0999, -4.3) -> (85.0999, -4.4617)
  arc A327 (85.0999, -4.3) -> (84.6999, -3.9) centre (84.6999, -4.3) ccw
  line L300 (84.5382, -3.9) -> (84.6999, -3.9)
  arc A328 (84.5382, -3.9) -> (84.3695, -3.9925) centre (84.5382, -4.1) ccw
  line L301 (84.211, -4.2413) -> (84.3695, -3.9925)
  arc A329 (83.9543, -4.3134) -> (84.211, -4.2413) centre (84.0423, -4.1338) ccw
  arc A330 (83.9543, -4.3134) -> (82.5454, -4.3134) centre (83.2499, -5.75) ccw
  arc A331 (82.2887, -4.2413) -> (82.5454, -4.3134) centre (82.4574, -4.1338) ccw
  line L302 (82.1302, -3.9925) -> (82.2887, -4.2413)
  arc A332 (82.1302, -3.9925) -> (81.9615, -3.9) centre (81.9615, -4.1) ccw
  line L303 (81.7999, -3.9) -> (81.9615, -3.9)
  arc A333 (81.7999, -3.9) -> (81.3999, -4.3) centre (81.7999, -4.3) ccw
  line L304 (81.3999, -4.4617) -> (81.3999, -4.3)
  arc A334 (81.3999, -4.4617) -> (81.4924, -4.6304) centre (81.5999, -4.4617) ccw
  line L305 (81.7411, -4.7889) -> (81.4924, -4.6304)
  arc A335 (81.8133, -5.0456) -> (81.7411, -4.7889) centre (81.6337, -4.9575) ccw
  arc A336 (81.8133, -5.0456) -> (81.8133, -6.4544) centre (83.2499, -5.75) ccw
  arc A337 (81.7411, -6.7112) -> (81.8133, -6.4544) centre (81.6337, -6.5425) ccw
  line L306 (81.4924, -6.8696) -> (81.7411, -6.7112)
  arc A338 (81.4924, -6.8696) -> (81.3999, -7.0383) centre (81.5999, -7.0383) ccw
  line L307 (81.3999, -7.2) -> (81.3999, -7.0383)
  arc A339 (81.3999, -7.2) -> (81.7999, -7.6) centre (81.7999, -7.2) ccw
  line L308 (81.9615, -7.6) -> (81.7999, -7.6)
  arc A340 (81.9615, -7.6) -> (82.1302, -7.5075) centre (81.9615, -7.4) ccw
  line L309 (82.2887, -7.2587) -> (82.1302, -7.5075)
  arc A341 (105.3134, -5.0454) -> (105.2413, -4.7887) centre (105.1338, -4.9574) ccw
  arc A342 (105.3134, -5.0454) -> (105.3134, -6.4543) centre (106.75, -5.7499) ccw
  arc A343 (105.2413, -6.711) -> (105.3134, -6.4543) centre (105.1338, -6.5423) ccw
  line L310 (104.9925, -6.8695) -> (105.2413, -6.711)
  arc A344 (104.9925, -6.8695) -> (104.9, -7.0382) centre (105.1, -7.0382) ccw
  line L311 (104.9, -7.1999) -> (104.9, -7.0382)
  arc A345 (104.9, -7.1999) -> (105.3, -7.5999) centre (105.3, -7.1999) ccw
  line L312 (105.4617, -7.5999) -> (105.3, -7.5999)
  arc A346 (105.4617, -7.5999) -> (105.6304, -7.5073) centre (105.4617, -7.3999) ccw
  line L313 (105.7888, -7.2586) -> (105.6304, -7.5073)
  arc A347 (106.0456, -7.1864) -> (105.7888, -7.2586) centre (105.9575, -7.366) ccw
  arc A348 (106.0456, -7.1864) -> (107.4544, -7.1864) centre (106.75, -5.7499) ccw
  arc A349 (107.7111, -7.2586) -> (107.4544, -7.1864) centre (107.5425, -7.366) ccw
  line L314 (107.8696, -7.5073) -> (107.7111, -7.2586)
  arc A350 (107.8696, -7.5073) -> (108.0383, -7.5999) centre (108.0383, -7.3999) ccw
  line L315 (108.2, -7.5999) -> (108.0383, -7.5999)
  arc A351 (108.2, -7.5999) -> (108.6, -7.1999) centre (108.2, -7.1999) ccw
  line L316 (108.6, -7.0382) -> (108.6, -7.1999)
  arc A352 (108.6, -7.0382) -> (108.5075, -6.8695) centre (108.4, -7.0382) ccw
  line L317 (108.2587, -6.711) -> (108.5075, -6.8695)
  arc A353 (108.1866, -6.4543) -> (108.2587, -6.711) centre (108.3662, -6.5423) ccw
  arc A354 (108.1866, -6.4543) -> (108.1866, -5.0454) centre (106.75, -5.7499) ccw
  arc A355 (108.2587, -4.7887) -> (108.1866, -5.0454) centre (108.3662, -4.9574) ccw
  line L318 (108.5075, -4.6302) -> (108.2587, -4.7887)
  arc A356 (108.5075, -4.6302) -> (108.6, -4.4615) centre (108.4, -4.4615) ccw
  line L319 (108.6, -4.2999) -> (108.6, -4.4615)
  arc A357 (108.6, -4.2999) -> (108.2, -3.8999) centre (108.2, -4.2999) ccw
  line L320 (108.0383, -3.8999) -> (108.2, -3.8999)
  arc A358 (108.0383, -3.8999) -> (107.8696, -3.9924) centre (108.0383, -4.0999) ccw
  line L321 (107.7111, -4.2411) -> (107.8696, -3.9924)
  arc A359 (107.4544, -4.3133) -> (107.7111, -4.2411) centre (107.5425, -4.1337) ccw
  arc A360 (107.4544, -4.3133) -> (106.0456, -4.3133) centre (106.75, -5.7499) ccw
  arc A361 (105.7888, -4.2411) -> (106.0456, -4.3133) centre (105.9575, -4.1337) ccw
  line L322 (105.6304, -3.9924) -> (105.7888, -4.2411)
  arc A362 (105.6304, -3.9924) -> (105.4617, -3.8999) centre (105.4617, -4.0999) ccw
  line L323 (105.3, -3.8999) -> (105.4617, -3.8999)
  arc A363 (105.3, -3.8999) -> (104.9, -4.2999) centre (105.3, -4.2999) ccw
  line L324 (104.9, -4.4615) -> (104.9, -4.2999)
  arc A364 (104.9, -4.4615) -> (104.9925, -4.6302) centre (105.1, -4.4615) ccw
  line L325 (105.2413, -4.7887) -> (104.9925, -4.6302)
  line L326 (55, -17.5) -> (110, -17.5)
  line L327 (110, 5) -> (110, -35)
  line L328 (110, -17.5) -> (95, -17.5)
  circle A365 centre (83.2499, -5.75) radius 1.6
  circle A366 centre (83.25, -29.2501) radius 1.6
  circle A367 centre (106.7501, -29.25) radius 1.6
  circle A368 centre (106.75, -5.7499) radius 1.6
  circle A369 centre (95, -17.5) radius 3.5
  point P0 (55, 39)
  point P1 (15, -17.5)
  point P2 (15, -17.5)
  point P3 (95, -17.5)
  point P4 (95, -17.5)
  dimension "d24" = 35
  dimension "d25" = 90
  dimension "d26" = 15
  constraints: 720 point on circle, 654 end point, 531 symmetric about line, 368 centre point, 8 coincident, 6 point on line, 4 concentric, 2 horizontal, 2 midpoint, 2 perpendicular, 1 vertical, 190 other
  measures "d24" distance of L161.start L161.end
  measures "d25" angle of L161 L162
  measures "d26" distance of L163.end L165.end